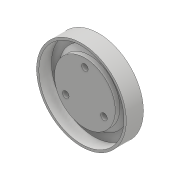
# Autodesk Inventor part: Arm - slew column C
Saved by Autodesk Inventor 2017 (Build 210142000, 142)
## iProperties
Created: 2017-06-18
Part Number: Arm - slew column C
Material: Generic
Document SubType Name: Modeling
Designer: Ali
Density: 1 g/cm^3
Appearance: Default
Author: Ali
Autodesk Inventor part; units mm, degrees
ref_plane "YZ Plane" through (0, 0, 0) normal (1, 0, 0) x (0, 1, 0)
ref_plane "XZ Plane" through (0, 0, 0) normal (0, 1, 0) x (-1, 0, 0)
ref_plane "XY Plane" through (0, 0, 0) normal (0, 0, 1) x (1, 0, 0)
sketch "Sketch1" plane through (0, 0, 0) normal (0, 1, 0) x (-1, 0, 0)
  circle A0 centre (0, 0) radius 20
  dimension "d0" = 40
  constraints: 1 centre point, 1 coincident
  measures "d0" diameter of A0
extrude "Extrusion1" add sketch "Sketch1" along normal blind 6
sketch "Sketch2" plane through (0, 6, 0) normal (0, 1, 0) x (1, 0, 0)
  circle A0 centre (0, 0) radius 29.5
  dimension "d3" = 59
  constraints: 1 centre point, 1 coincident
  measures "d3" diameter of A0
extrude "Extrusion2" add sketch "Sketch2" along normal blind 3
sketch "Sketch3" plane through (0, 6, 0) normal (0, -1, 0) x (1, 0, 0)
  circle A0 centre (0, 0) radius 29.5 projected
  circle A1 centre (0, 0) radius 28
  dimension "d6" = 56
  constraints: 1 centre point, 1 coincident
  measures "d6" diameter of A1
extrude "Extrusion3" add sketch "Sketch3" along normal blind 8.3
sketch "Sketch4" plane through (0, 9, 0) normal (0, 1, 0) x (1, 0, 0)
  circle A0 centre (0, 0) radius 14.5 construction
  line L0 (0, 0) -> (0, -14.5) construction
  point P0 (12.5574, 7.25)
  point P1 (-12.5574, 7.25)
  dimension "d9" = 29
  dimension "d12" = 360
  constraints: 2 coincident, 2 end point, 1 vertical, 1 vertical alignment, 6 other
hole "Hole1" at (0, 9, 14.5) at (12.5574, 9, -7.25) at (-12.5574, 9, -7.25) direction (0, -1, 0) diameter 4.3 end through all
chamfer "Chamfer1" distance 3 angle 45 1 edges at (20, 6, 0)
sketch "Sketch5" plane through (0, 9, 0) normal (0, 1, 0) x (1, 0, 0)
  circle A0 centre (0, -14.5) radius 2.15 projected
  circle A1 centre (-12.5574, 7.25) radius 2.15 projected
  circle A2 centre (12.5574, 7.25) radius 2.15 projected
  circle A3 centre (0, -14.5) radius 4.25
  circle A4 centre (-12.5574, 7.25) radius 4.25
  circle A5 centre (12.5574, 7.25) radius 4.25
  point P0 (0, 0)
  dimension "d24" = 8.5
  dimension "d25" = 8.5
  dimension "d26" = 8.5
  constraints: 3 centre point, 3 coincident
  measures "d24" diameter of A3
  measures "d25" diameter of A5
  measures "d26" diameter of A4
extrude "Extrusion4" cut sketch "Sketch5" against normal blind 5
equation "\"d25\" = d24"
equation "\"d26\" = d24"
body "Solid1"
